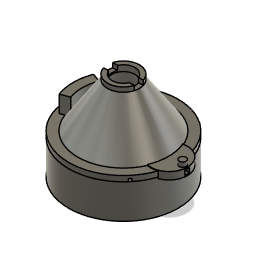
Cheerioboat triple channel v2 (Autodesk Fusion 360 design; units mm, degrees)
Autodesk Fusion 360 part; units mm, degrees
note: some values were not read from the file. Set by a fixed rule: which sketch regions a step uses.
sketch "Boat silouette" plane through (0, 0, 0) normal (1, 0, 0) x (0, 0, -1)
  line L0 (0, 0) -> (-12, 0)
  line L1 (-12, 0) -> (-12, 8.7)
  line L2 (-12, 8.7) -> (-10, 8.7)
  line L3 (0, 0) -> (0, 1)
  line L4 (0, 1) -> (-11, 1)
  line L5 (-3.5, 19.5) -> (-2.5, 19.5)
  line L6 (-3.5, 19.5) -> (-3.5, 18.5)
  line L7 (-10, 8.7) -> (-3.5, 18.5)
  line L8 (-2.5, 19.5) -> (-2.5, 18.1985)
  line L9 (-2.5, 18.1985) -> (-9.596, 7.5)
  line L10 (-9.596, 7.5) -> (0, 7.5)
  line L11 (0, 7.5) -> (0, 6.5)
  line L12 (0, 6.5) -> (-11, 6.5)
  line L13 (-11, 6.5) -> (-11, 1)
  line L14 (-9.596, 7.5) -> (-12, 7.5)
  dimension "d2" = 12
  dimension "d3" = 8.7
  dimension "d4" = 2
  dimension "d5" = 1
  dimension "d6" = 11
  dimension "d10" = 1
  dimension "d11" = 1
  dimension "d13" = 1
  dimension "d14" = 19.5
  dimension "d15" = 2.5
  dimension "d19" = 1
  dimension "d20" = 1.2
  constraint coincident L0.start L3.start
  constraint horizontal L0
  constraint perpendicular L0 L1
  constraint perpendicular L1 L2
  constraint perpendicular L0 L3
  constraint perpendicular L3 L4
  constraint horizontal L5
  constraint perpendicular L5 L6
  constraint perpendicular L5 L8
  constraint parallel L7 L9
  constraint perpendicular L11 L12
  constraint coincident L1 L14.end
  constraint perpendicular L1 L14
  measures "d2" distance of L0.start L0.end
  measures "d3" distance of L0.end L1.end
  measures "d4" distance of L1.end L2.end
  measures "d5" distance of L0.start L3.end
  measures "d6" distance of L3.end L4.end
  measures "d10" distance of L5.start L6.end
  measures "d11" distance of L7 L9
  measures "d13" distance of L6 L8
  measures "d14" distance of L0 L5
  measures "d15" distance of L3 L8
  measures "d19" distance of L10.end L11.end
  measures "d20" distance of L2 L10
sketch "Tracking cap slot" plane through (0, 0, 0) normal (1, 0, 0) x (0, 0, -1)
  line L0 (1, 19.5) -> (-1, 19.5)
  line L1 (-1, 19.5) -> (-1, 18.5)
  line L2 (-1, 18.5) -> (1, 18.5)
  line L3 (1, 18.5) -> (1, 19.5)
  line L4 (1, 19.5) -> (-1, 18.5) construction
  line L5 (-1, 19.5) -> (1, 18.5) construction
  point P0 (0, 19)
  dimension "d17" = 2
  dimension "d18" = 1
  constraint horizontal L0
  constraint perpendicular L0 L1
  constraint parallel L0 L2
  constraint parallel L1 L3
  constraint coincident L4 P0
  constraint coincident L5 P0
  measures "d17" distance of L1.end L2.end
  measures "d18" distance of L0.end L1.end
sketch "Single slit hole" plane through (0, 0, 0) normal (1, 0, 0) x (0, 0, -1)
  line L0 (0.25, 8) -> (-0.25, 8)
  line L1 (-0.25, 8) -> (-0.25, 7.5)
  line L2 (-0.25, 7.5) -> (0.25, 7.5)
  line L3 (0.25, 7.5) -> (0.25, 8)
  line L4 (0.25, 8) -> (-0.25, 7.5) construction
  line L5 (-0.25, 8) -> (0.25, 7.5) construction
  point P0 (0, 7.75)
  dimension "d21" = 0.5
  dimension "d22" = 0.5
  constraint horizontal L0
  constraint perpendicular L0 L1
  constraint parallel L0 L2
  constraint parallel L1 L3
  constraint coincident L4 P0
  constraint coincident L5 P0
  measures "d21" distance of L1.end L2.end
  measures "d22" distance of L0.end L1.end
revolve "Revolve5" add sketch "Boat silouette" angle 360 about axis through (0, 1.75, 0) along (0, 1, 0) contours L0 L1 L3 L4 L10 L11 L12 L13 L14 makes body 1
revolve "Revolve6" add sketch "Boat silouette" angle 360 about axis through (0, 1.75, 0) along (0, 1, 0) separate body contours L1 L2 L5 L6 L7 L8 L9 L14 makes body 2
sketch "Nozzle" plane through (0, 7.5, 0) normal (0, 1, 0) x (-1, 0, 0)
  circle A0 centre (0, 0) radius 12
  circle A1 centre (0, 0) radius 12
  circle A2 centre (0, 0) radius 10
  circle A3 centre (-10, 0) radius 4
  circle A4 centre (-10, 0) radius 4.02
  line L0 (-6.0314, 0.5) -> (-13.9686, 0.5)
  line L1 (-6.0314, -0.5) -> (-13.9686, -0.5)
  arc A5 (-9.1925, 7.7135) -> (-9.1925, -7.7135) centre (0, 0) ccw
  line L2 (0, 0) -> (-9.1925, 7.7135) construction
  line L3 (0, 0) -> (-9.1925, -7.7135) construction
  line L4 (-9.1925, 7.7135) -> (0, 0)
  line L5 (-9.1925, -7.7135) -> (0, 0)
  line L6 (-7.1955, 5.6461) -> (-6.8099, 6.1058)
  line L7 (-6.8099, 6.1058) -> (-9.874, 8.6769)
  line L8 (-9.874, 8.6769) -> (-10.2597, 8.2173)
  line L9 (-10.2597, 8.2173) -> (-7.1955, 5.6461)
  line L10 (-6.6121, -5.9398) -> (-6.9978, -5.4802)
  line L11 (-6.9978, -5.4802) -> (-10.062, -8.0514)
  line L12 (-6.6121, -5.9398) -> (-9.6763, -8.511)
  line L13 (-9.6763, -8.511) -> (-10.062, -8.0514)
  dimension "d47" = 24
  dimension "d48" = 20
  dimension "d49" = 8
  dimension "d50" = 0.02
  dimension "d51" = 1
  dimension "d71" = 80
  dimension "d72" = 0.6
  dimension "d73" = 0.3
  dimension "d74" = 0.6
  dimension "d75" = 4
  dimension "d76" = 4
  dimension "d77" = 4
  dimension "d78" = 0.3
  constraint coincident A0.centre A1.centre
  constraint coincident A2 A3.centre
  constraint concentric A3 A4
  constraint coincident A3 L0.start
  constraint coincident A3 L0.end
  constraint horizontal L0
  constraint coincident A3 L1.start
  constraint coincident A3 L1.end
  constraint parallel L0 L1
  constraint equal L0 L1
  constraint coincident A1 A5.end
  constraint perpendicular L4 L6
  constraint perpendicular L6 L7
  constraint perpendicular L7 L8
  constraint perpendicular L6 L9
  constraint perpendicular L5 L10
  constraint perpendicular L10 L11
  constraint perpendicular L10 L12
  measures "d47" diameter of A1
  measures "d48" diameter of A2
  measures "d49" diameter of A3
  measures "d50" distance of A3 A4
  measures "d51" distance of L0 L1
  measures "d71" angle of L2 L3
  measures "d72" distance of L7 L9
  measures "d73" distance of L2 L9
  measures "d74" distance of L10.start L10.end
  measures "d75" distance of L10.end L11.end
  measures "d76" distance of L10.start L12.end
  measures "d77" distance of L6 L8
  measures "d78" distance of L5 L12
extrude "Extrude7" cut sketch "Nozzle" along normal blind 1.32 and the other way blind 0.32 contours A0 A1 A2 A3 A4 A5 | A0 A1 A3 A4 A5 | A0 A1 A2 A3 A4 A5 | A0 A1 A2 A3 L0 A5 | A0 A1 A3 L0 A5 | A2 A3 A4 | A0 A1 A3 L1 A5 | A0 A1 A2 A3 L1 A5 | A0 A1 A2 L0 L1 A5 | A0 A1 A3 L0 L1 A5 | A2 A3 L0 | A2 A3 L1 | A2 A3 L0 L1 bodies 2 1
extrude "Extrude8" add sketch "Nozzle" along normal blind 1.3 and the other way blind 0.3 separate body contours A0 A1 A2 A3 A4 L0 A5 | A0 A1 A3 A4 L0 A5 | A0 A1 A3 A4 L1 A5 | A0 A1 A2 A3 A4 L1 A5 | A0 A1 A2 L0 L1 A5 | A0 A1 A3 A4 L0 L1 A5 | A2 A3 A4 L0 | A2 A3 A4 L1 | A2 A3 A4 L0 L1 makes body 3
extrude "Extrude9" cut sketch "Nozzle" along normal blind 1 contours A0 A1 A2 L0 L1 A5 | A0 A1 A3 L0 L1 A5 | A2 A3 L0 L1 bodies 3
extrude "Extrude10" cut sketch "Tracking cap slot" along normal mid plane 30 bodies 2
sketch "Pin" plane through (0, 8.8, 0) normal (0, 1, 0) x (-1, 0, 0)
  circle A0 centre (-10, 0) radius 4
  circle A1 centre (-10, 0) radius 4
  circle A2 centre (-13, 0) radius 0.75
  dimension "d64" = 1.5
  constraint concentric A0 A1
  measures "d64" diameter of A2
extrude "Extrude11" add sketch "Pin" along normal blind 1 contours A2 bodies 3
sketch "Sketch10" plane through (0, 8.7, 0) normal (0, 1, 0) x (-1, 0, 0)
  arc A0 (-11.392, -3.7713) -> (-9.192, -3.938) centre (-10, 0) ccw
  arc A1 (-11.392, -3.7713) -> (-11.392, 3.7713) centre (0, 0) ccw
  arc A2 (-9.192, 3.938) -> (-11.392, 3.7713) centre (-10, 0) ccw
  arc A3 (-9.192, -3.938) -> (-9.192, 3.938) centre (0, 0) ccw
  circle A4 centre (0, 0) radius 10
  circle A5 centre (0, 0) radius 11
  circle A6 centre (0, 0) radius 9
  line L0 (0, 0) -> (11, 0)
  line L1 (0, 0) -> (10.3366, 3.7622)
  line L2 (0, 0) -> (10.3366, -3.7622)
  dimension "d67" = 18
  dimension "d68" = 20
  constraint coincident A1.centre A3.centre
  constraint concentric A5 A6
  constraint coincident A5 L0.end
  constraint horizontal L0
  constraint coincident A5 L1.end
  constraint symmetric L0 A1.centre A3.centre
  constraint symmetric L0 L1.end L2.end
  measures "d67" diameter of A6
  measures "d68" angle of L0 L1
extrude "Extrude12" add sketch "Sketch10" along normal blind 3.7 separate body contours A3 A4 A5 L0 L2 | A3 A4 A6 L0 L2 | A3 A4 A5 L0 L1 | A3 A4 A6 L0 L1 makes body 4
extrude "Extrude13" cut sketch "Nozzle" along normal blind 0.6 contours A0 A1 A2 L4 L7 | A0 A1 A5 L7 L8 L9 | A0 A1 A5 L11 L12 L13 | A0 A1 A2 L5 L12 | A0 A1 A2 A5 L4 L9 | A2 L4 L6 L7 | A0 A1 A2 A5 L5 L11 | A2 L5 L10 L12 | A2 L4 L6 L9 | A2 L5 L10 L11 bodies 2
named bodies: "Boat bottom", "Boat fuel containter", "Nozzle", "Counterbalance"
